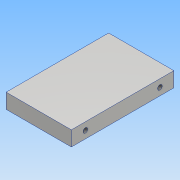
# Autodesk Inventor part: Pancake_Floor Piece
Saved by Autodesk Inventor 2018.1 (Build 221171000, 171)
## iProperties
Created: 2019-02-28
Part Number: Pancake_Floor Piece
Material: Aluminum 6061
Document SubType Name: Modeling
Designer: James
Density: 2.7 g/cm^3
Appearance: Aluminum - Flat
Author: James
Autodesk Inventor part; units mm, degrees
ref_plane "YZ Plane" through (0, 0, 0) normal (1, 0, 0) x (0, 1, 0)
ref_plane "XZ Plane" through (0, 0, 0) normal (0, 1, 0) x (-1, 0, 0)
sketch "Sketch1" plane through (0, 0, 0) normal (0, 0, 1) x (1, 0, 0)
  line L0 (0, 0) -> (35, 0)
  line L1 (35, 0) -> (35, 55)
  line L2 (35, 55) -> (0, 55)
  line L3 (0, 55) -> (0, 0)
  dimension "d0" = 35
  dimension "d1" = 55
  constraints: 8 end point, 2 parallel, 1 horizontal, 1 perpendicular
  measures "d0" distance of L2.end L1.end
  measures "d1" distance of L1.end L0.end
extrude "Extrusion1" add sketch "Sketch1" along normal mid plane 8
sketch "Sketch2" plane through (35, 0, 4) normal (1, 0, 0) x (0, 0, -1)
  line L0 (8, 55) -> (0, 55) projected
  point P0 (4, 0)
  point P1 (4, 7.5)
  point P2 (4, 47.5)
  point P3 (4, 55)
  dimension "d4" = 7.5
  dimension "d5" = 7.5
  dimension "d6" = 40
  constraints: 2 vertical alignment, 1 midpoint
  measures "d4" distance from line of L0 point (4, 47.5)
  measures "d5" distance of point (4, 0) point (4, 7.5)
  measures "d6" distance of point (4, 47.5) point (4, 7.5)
hole "Hole1" at (35, 7.5, 0) at (35, 47.5, 0) direction (-1, 0, 0) diameter 2.459 depth 8.8 tip angle 118 thread size "M3x0.5" class "6H" standard "ANSI Metric M Profile"
ref_plane "Work Plane1" through (17.5, 0, 4) normal (1, 0, 0) x (0, 0, -1)
mirror "Mirror1" about plane through (17.5, 0, 4) normal (1, 0, 0) of "Hole1"
equation "\"d5\" = d4"
body "Solid1"
